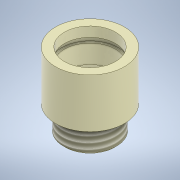
# Autodesk Inventor part: Heated tube-transfer tube connector
Saved by Autodesk Inventor 2020.3 (Build 243373000, 373)
## iProperties
Created: 2020-08-24
Part Number: Heated tube-transfer tube connector
Material: Polypropylene
Document SubType Name: Modeling
Designer: Bruno
Density: 0.899 g/cm^3
Appearance: Smooth - Ash
Author: Bruno
Autodesk Inventor part; units mm, degrees
ref_plane "YZ Plane" through (0, 0, 0) normal (1, 0, 0) x (0, 1, 0)
ref_plane "XZ Plane" through (0, 0, 0) normal (0, 1, 0) x (-1, 0, 0)
ref_plane "XY Plane" through (0, 0, 0) normal (0, 0, 1) x (1, 0, 0)
sketch "Sketch1" plane through (0, 0, 0) normal (0, 0, 1) x (1, 0, 0)
  line L0 (0, 0) -> (-13.5, 0)
  line L1 (-13.5, 0) -> (-13.5, 13)
  line L2 (-13.5, 13) -> (-17.5, 13)
  line L3 (-17.5, 13) -> (-17.5, 38)
  line L4 (-17.5, 38) -> (-13, 38)
  line L5 (-13, 38) -> (-13, 33)
  line L6 (-13, 33) -> (-14.35, 33)
  line L7 (-14.35, 33) -> (-14.35, 30.5)
  line L8 (-14.35, 30.5) -> (-13, 30.5)
  line L9 (-13, 30.5) -> (-13, 18)
  line L10 (-13, 18) -> (-10, 18)
  line L11 (-10, 18) -> (-10, 0)
  line L12 (0, 0) -> (0, 38)
  dimension "d0" = 13.5
  dimension "d1" = 13
  dimension "d2" = 4
  dimension "d3" = 25
  dimension "d4" = 4.5
  dimension "d5" = 5
  dimension "d6" = 1.35
  dimension "d7" = 2.5
  dimension "d8" = 12.5
  dimension "d9" = 3
  constraints: 26 end point, 10 perpendicular, 3 point on line, 1 horizontal, 1 vertical
  measures "d0" distance of L0.start L0.end
  measures "d1" distance of L0.end L1.end
  measures "d2" distance of L1.end L2.end
  measures "d3" distance of L2.end L3.end
  measures "d4" distance of L3.end L4.end
  measures "d5" distance of L4.end L5.end
  measures "d6" distance of L5.end L6.end
  measures "d7" distance of L6.end L7.end
  measures "d8" distance of L8.end L9.end
  measures "d9" distance of L9.end L10.end
revolve "Revolution1" add sketch "Sketch1" angle 360 about axis through (0, 0, 0) along (0, 1, 0)
fillet "Fillet1" radius 2 1 edges at (13.5, 13, 0)
chamfer "Chamfer1" distance 3 angle 45 1 edges at (13, 18, 0)
chamfer "Chamfer2" distance 1 angle 45 1 edges at (13.5, 0, 0)
thread "Thread1" size "M27x3" class "6g" standard "ANSI Metric M Profile" full length
body "Solid1"
